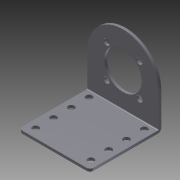
# Autodesk Inventor part: HD-BK-IG
Saved by Autodesk Inventor 2012 (Build 160160000, 160)
## iProperties
Created: 2013-07-13
Part Number: HD-BK-IG
Material: Galvanized Steel
Document SubType Name: Sheet Metal
Designer: joe_000
Density: 7.85 g/cm^3
Sheet Metal Rule: Default
Mass: 29.4767 g
Surface Area: 56.306 cm^2
Volume: 3.75499 cm^3
d46: 4.000 ul
HoleSpacing: 31.000 mm
Thickness: 1.500 mm
MotorCenterOffset: 20.500 mm
Author: joe_000
Autodesk Inventor part; units mm, degrees
ref_plane "YZ Plane" through (0, 0, 0) normal (1, 0, 0) x (0, 1, 0)
ref_plane "XZ Plane" through (0, 0, 0) normal (0, 1, 0) x (-1, 0, 0)
ref_plane "XY Plane" through (0, 0, 0) normal (0, 0, 1) x (1, 0, 0)
sketch "Sketch1" plane through (0, 0, 0) normal (0, 0, 1) x (1, 0, 0)
  line L0 (20, 0) -> (20, -20.5)
  line L1 (20, -20.5) -> (-20, -20.5)
  line L2 (-20, -20.5) -> (-20, 0)
  arc A0 (20, 0) -> (-20, 0) centre (0, 0) ccw
  circle A1 centre (0, 0) radius 10.5
  dimension "d1" = 40
  dimension "d4" = 20
  dimension "d5" = 20.5
  dimension "d7" = 21
  dimension "d8" = 20
  dimension "MotorCenterOffset" = 20.5
  measures "d1" distance of L0.end L1.end
  measures "d4" radius of A0
  measures "d5" distance of L0.start L0.end
  measures "d7" diameter of A1
  measures "d8" distance from line of L2 A0.centre
  measures "MotorCenterOffset" distance from line of A0.centre L1
extrude "Plate1" add sketch "Sketch1" along normal blind 1.5
sketch "Sketch3" plane through (20, -19, 0) normal (0, -1, 0) x (1, 0, 0)
  line L0 (-40, 0) -> (0, 0)
  line L1 (0, 0) -> (0, 40)
  line L2 (0, 40) -> (-40, 40)
  line L3 (-40, 40) -> (-40, 0)
  constraints: 8 end point
edge flange "Flange1" height 40 angle 90 thickness 1.5 bend radius 0.5 thickness toward (0, -1, 0) relief tear relief width 1.5 relief depth 0.75 edges at (0, -20.5, 1.5) wall of the first edge with corners at (-20, -19, 0) (20, -19, 0) (20, -19, 40) (-20, -19, 40)
bend "Bend1"
corner "Corner1"
fillet "Corner Round1" radius 2 1 edges at (-20, -19.75, 40)
fillet "Corner Round1" radius 2 1 edges at (20, -19.75, 40)
sketch "Sketch4" plane through (-20, -19, 2) normal (0, 1, 0) x (1, 0, 0)
  line L0 (2, -38) -> (38, -38) projected
  line L1 (0, -36) -> (0, 0) projected
  line L2 (0, -33) -> (4.5, -33)
  line L3 (4.5, -33) -> (4.5, -38)
  point P0 (20, 2)
  dimension "d43" = 4.5
  dimension "d44" = 5
  constraints: 4 end point, 2 perpendicular, 2 point on line
  measures "d43" distance of L2.start L2.end
  measures "d44" distance of L2.end L3.end
hole "Hole2" at (-15.5, -19, 35) direction (0, -1, 0) diameter 3.5 end through all
pattern_linear "Rectangular Pattern2" count 4 spacing 10 along (0, 0, -1) count 2 spacing 31 along (1, 0, 0) of "Hole2"
sketch "Sketch5" plane through (0, 0, 1.5) normal (0, 0, 1) x (1, 0, 0)
  line L0 (-20, -18.5) -> (-20, 0) projected
  circle A0 centre (0, 0) radius 10.5 projected
  line L1 (0, 0) -> (9.1924, 9.1924)
  circle A1 centre (0, 0) radius 13
  line L2 (0, 0) -> (13, 0)
  circle A2 centre (9.1924, 9.1924) radius 1.75
  dimension "d59" = 26
  dimension "d60" = 45
  dimension "d61" = 3.5
  constraints: 4 end point, 2 centre point, 2 coincident, 2 point on circle, 1 perpendicular
  measures "d59" diameter of A1
  measures "d60" angle of L2 L1
  measures "d61" diameter of A2
hole "Hole3" at (9.1924, 9.1924, 1.5) direction (0, 0, -1) diameter 3.5 end through all
pattern_circular "Circular Pattern1" count 4 over 360 about axis through (0, 0, 0) along (0, 0, 1) of "Hole3"
equation "\"d50\" = Thickness"
equation "\"d12\" = BendReliefWidth"
equation "\"d13\" = BendReliefDepth"
equation "\"d14\" = MinimumRemnant"
equation "\"d15\" = BendRadius"
equation "\"d19\" = CornerReliefSize"
equation "\"d20\" = GapSize"
equation "\"d21\" = JacobiRadiusSize"
equation "\"BendRadius\" = Thickness"
equation "\"BendReliefWidth\" = Thickness"
equation "\"BendReliefDepth\" = 0.5 * Thickness"
equation "\"CornerReliefSize\" = 4 * Thickness"
equation "\"MinimumRemnant\" = 2 * Thickness"
equation "\"TransitionRadius\" = BendRadius"
equation "\"JacobiRadiusSize\" = BendRadius"
equation "\"GapSize\" = Thickness"
equation "\"d10\" = BendRadius"
equation "\"Thickness\" = 1.5"
body "Solid1"
